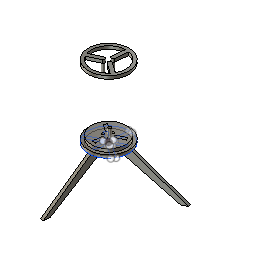
Tower Launcher (Autodesk Fusion 360 design; units mm, degrees)
Autodesk Fusion 360 part; units mm, degrees
sketch "main" plane through (0, 0, 0) normal (1, 0, 0) x (0, 0, -1)
  circle A0 centre (-0.121, 13.4986) radius 6
  circle A1 centre (0, 0) radius 55
  circle A2 centre (-0.121, 13.4986) radius 5
  circle A3 centre (-0.001, -0.0014) radius 65
  line L0 (5.879, 13.4986) -> (5.879, 64.7321)
  line L1 (-6.121, 13.4986) -> (-6.121, 64.7099)
  circle A4 centre (-11.6323, -6.8553) radius 5
  line L2 (-8.6323, -12.0514) -> (-52.9826, -37.6571)
  line L3 (-14.6323, -1.6591) -> (-59.0018, -27.2759)
  circle A5 centre (-11.6323, -6.8553) radius 6
  circle A6 centre (11.7504, -6.6475) radius 5
  line L4 (14.7504, -1.4513) -> (59.1006, -27.0569)
  line L5 (8.7504, -11.8436) -> (53.1199, -37.4604)
  circle A7 centre (11.7504, -6.6475) radius 6
  line L6 (4.999, -44.3259) -> (-5.001, -44.3259)
  line L7 (-5.001, -44.3259) -> (-5.001, -14.3259)
  line L8 (-5.001, -14.3259) -> (4.999, -14.3259)
  line L9 (4.999, -14.3259) -> (4.999, -44.3259)
  line L10 (9.9044, 11.491) -> (35.8852, 26.491)
  line L11 (40.8852, 17.8307) -> (14.9044, 2.8307)
  line L12 (14.9044, 2.8307) -> (9.9044, 11.491)
  line L13 (35.8852, 26.491) -> (40.8852, 17.8307)
  line L14 (-14.9063, 2.8307) -> (-40.8871, 17.8307)
  line L15 (-35.8871, 26.491) -> (-9.9063, 11.491)
  line L16 (-9.9063, 11.491) -> (-14.9063, 2.8307)
  line L17 (-40.8871, 17.8307) -> (-35.8871, 26.491)
  circle A8 centre (-0.121, 13.4986) radius 4
  circle A9 centre (-11.6323, -6.8553) radius 4
  circle A10 centre (11.7504, -6.6475) radius 4
  dimension "d7" = 12
  dimension "d8" = 13.5
  dimension "d11" = 110
  dimension "d19" = 10
  dimension "d27" = 130
  dimension "d70" = 360
  dimension "d77" = 30
  dimension "d79" = 360
  dimension "d84" = 10
  dimension "d106" = 5
  dimension "d114" = 8
  constraint coincident A1.centre origin
  constraint coincident A0 L0.start
  constraint coincident A3 L0.end
  constraint tangent A0 L0
  constraint vertical L0
  constraint coincident A0 L1.start
  constraint coincident A3 L1.end
  constraint tangent A0 L1
  constraint parallel L0 L1
  constraint horizontal L6
  constraint vertical L7
  constraint horizontal L8
  constraint vertical L9
  constraint concentric A0 A2
  constraint concentric A0 A8
  measures "d7" diameter of A0
  measures "d8" vertical distance of A0.centre A3.centre
  measures "d11" diameter of A1
  measures "d19" diameter of A2
  measures "d27" diameter of A3
  measures "d77" distance of L6.start L8.end
  measures "d84" distance of L6.start L6.end
  measures "d106" horizontal distance of A3.centre L8.end
  measures "d114" diameter of A8
extrude "base" add sketch "main" along normal blind 10 contours A0 | A0 A1 L0 L1 L2 L3 A5 L4 L5 A7 | A0 A1 L0 L1 | A1 A3 L0 L4 | A1 A3 L0 L1 | A1 A3 L1 L3 | A1 L2 L3 A5 | A1 A3 L2 L3 | A1 A3 L4 L5 | A1 L4 L5 A7 | A1 A3 L2 L5 | A5 | A7 | A2 | A4 | A6 | A8 | A9 | A10 makes body 1
sketch "leg" plane through (0, 0, 5.001) normal (0, 0, -1) x (-1, 0, 0)
  line L0 (0, -44.3259) -> (0, -14.3259)
  line L1 (0, -14.3259) -> (-10, -14.3259)
  line L2 (128.5575, -197.5348) -> (128.5575, -177.5348)
  line L3 (0, -14.3259) -> (-20, -14.3259)
  line L4 (-20, -44.3259) -> (-20, -14.3259)
  line L5 (0, -9.3259) -> (128.5575, -177.5348)
  line L6 (0, -44.3259) -> (0, -49.3259)
  line L7 (0, -49.3259) -> (128.5575, -197.5348)
  line L8 (-20, -44.3259) -> (0, -44.3259)
  line L9 (0, -9.3259) -> (0, -14.3259)
  line L10 (0, -44.3259) -> (0, -14.3259)
  line L11 (0, -14.3259) -> (-10, -14.3259)
  line L12 (-10, -14.3259) -> (-10, -44.3259)
  line L13 (-10, -44.3259) -> (0, -44.3259)
  dimension "d81" = 200
  dimension "d83" = 20
  dimension "d89" = 20
  dimension "d103" = 5
  constraint coincident L0.start L6.start
  constraint vertical L2
  constraint coincident L0.end L1.start
  constraint perpendicular L3 L4
  constraint perpendicular L6 L8
  measures "d81" distance of L0.start L2.start
  measures "d83" distance of L2.start L2.end
  measures "d89" distance of L0.end L3.end
  measures "d103" distance of L0.end L5.start
extrude "leg (1)" add sketch "leg" along normal blind 10 separate body makes body 2
pattern_circular "all legs" count 3 over 360 about axis through (1.75, 0, 0) along (1, 0, 0) of "leg (1)" makes body 3 makes body 4
extrude "lower_mount" add sketch "main" along normal blind 10 from surface at 10 separate body contours A0 | A0 A1 L0 L1 L2 L3 A5 L4 L5 A7 | A0 A1 L0 L1 | A1 L2 L3 A5 | A1 L4 L5 A7 | A5 | A7 | A2 | A4 | A6 | A8 | A9 | A10 makes body 5
extrude "lower_pegs" cut sketch "main" against normal through all from surface at 20 contours A8 | A9 | A10 bodies 5
extrude "upper_mount" add sketch "main" along normal blind 10 from surface at 220 separate body contours A0 | A0 A1 L0 L1 | A1 A3 L0 L4 | A1 A3 L0 L1 | A1 A3 L1 L3 | A1 L2 L3 A5 | A1 A3 L2 L3 | A1 A3 L4 L5 | A1 L4 L5 A7 | A1 A3 L2 L5 | A5 | A7 | A2 | A4 | A6 | A8 | A9 | A10 makes body 6
extrude "upper_pegs" add sketch "main" against normal blind 30 from surface at 220 contours A2 | A4 | A6 | A8 | A9 | A10 bodies 6
copy_body "Body->Comp1" bodies 1 removing the originals makes body 7 in component "base"
copy_body "Body->Comp2" bodies 5 removing the originals makes body 8 in component "mount_lower"
copy_body "Body->Comp4" bodies 2 removing the originals makes body 9 in component "leg1"
copy_body "Body->Comp5" bodies 3 removing the originals makes body 10 in component "leg2"
copy_body "Body->Comp6" bodies 4 removing the originals makes body 11 in component "leg3"
copy_body "Body->Comp7" bodies 6 removing the originals makes body 12 in component "mount_upper"
extrude "Extrude1" add sketch "main" along normal blind 30 from surface at 20 separate body contours A4 makes body 13 in component "sleeve"
component "base" placed x (1, 0, 0) y (0, 1, 0) z (0, 0, 1) at (0, 0, 0)
component "mount_lower" placed x (1, 0, 0) y (0, 1, 0) z (0, 0, 1) at (0, 0, 0)
component "leg1" placed x (1, 0, 0) y (0, 1, 0) z (0, 0, 1) at (0, 0, 0)
component "leg2" placed x (1, 0, 0) y (0, 1, 0) z (0, 0, 1) at (0, 0, 0)
component "leg3" placed x (1, 0, 0) y (0, 1, 0) z (0, 0, 1) at (0, 0, 0)
component "mount_upper" placed x (1, 0, 0) y (0, 1, 0) z (0, 0, 1) at (0, 0, 0)
component "sleeve" placed x (1, 0, 0) y (0, 1, 0) z (0, 0, 1) at (0, 0, 0)
equation "d7 = tube_od"
equation "d8 = body_dia / 2 + tube_od / 2"
equation "d19 = tube_id"
equation "body_dia = 15 mm"
equation "tube_od = 12 mm"
equation "tube_id = 10 mm"
named bodies: "base", "leg1", "leg2", "leg3", "mount_lower", "mount_upper", "sleeve"
